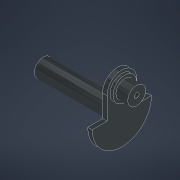
# Autodesk Inventor part: P015-Vilbrequin
Saved by Autodesk Inventor 2021.3 (Build 253353000, 353)
## iProperties
Created: 2022-04-01
Part Number: P015-Vilbrequin
Material: Iron, Gray
Document SubType Name: Modeling
Designer: remi
Density: 7.15 g/cm^3
Appearance: Iron Gray
Mass: 76.739 g
Surface Area: 54.5385 cm^2
Volume: 10.7327 cm^3
Author: remi
Autodesk Inventor part; units mm, degrees
ref_plane "YZ Plane" through (0, 0, 0) normal (1, 0, 0) x (0, 1, 0)
ref_plane "XZ Plane" through (0, 0, 0) normal (0, 1, 0) x (-1, 0, 0)
ref_plane "XY Plane" through (0, 0, 0) normal (0, 0, 1) x (1, 0, 0)
sketch "Sketch2" plane through (0, 0, 0) normal (1, 0, 0) x (0, 1, 0)
  arc A0 (-20, 0) -> (20, 0) centre (0, 0) ccw
  line L0 (-20, 0) -> (-10, 0)
  line L1 (-10, 0) -> (-10, 15)
  line L2 (20, 0) -> (10, 0)
  line L3 (10, 0) -> (10, 15)
  arc A1 (10, 15) -> (-10, 15) centre (0, 15) ccw
  dimension "d1" = 20
  dimension "d2" = 15
  dimension "d3" = 20
  constraints: 8 end point, 4 horizontal alignment, 4 point on circle, 2 centre point, 2 horizontal, 2 perpendicular, 1 coincident, 1 collinear
  measures "d1" distance between parallel lines of L3 L1
  measures "d2" distance of L2.end L3.end
  measures "d3" radius of A0
extrude "Extrusion1" add sketch "Sketch2" along normal blind 3
sketch "Sketch10" plane through (0, 0, 0) normal (-1, 0, 0) x (0, 0, 1)
  circle A0 centre (0, 0) radius 6
  dimension "d25" = 12
  constraints: 1 centre point, 1 coincident
  measures "d25" diameter of A0
extrude "Extrusion8" add sketch "Sketch10" along normal blind 50
sketch "Sketch11" plane through (3, 0, 0) normal (1, 0, 0) x (0, 0, -1)
  circle A0 centre (-15, 0) radius 6
  circle A1 centre (-15, 0) radius 8
  arc A2 (0, -20) -> (0, 20) centre (0, 0) ccw projected
  line L0 (0, 20) -> (0, 10) projected
  line L1 (0, 10) -> (-15, 10) projected
  arc A3 (-15, 10) -> (-15, -10) centre (-15, 0) ccw projected
  line L2 (-15, -10) -> (0, -10) projected
  line L3 (0, -10) -> (0, -20) projected
  dimension "d29" = 12
  dimension "d32" = 2
  constraints: 2 centre point, 2 coincident, 1 horizontal alignment
  measures "d29" diameter of A0
  measures "d32" radial gap between concentric circles of A1 A0
extrude "Extrusion9" add sketch "Sketch11" along normal blind 10 contours A0
extrude "Extrusion10" add sketch "Sketch11" along normal blind 2 contours A1
sketch "Sketch12" plane through (13, 0, 15) normal (1, 0, 0) x (0, 0, -1)
  circle A0 centre (0, 0) radius 6 construction
  point P0 (15, 0)
  constraints: 1 coincident
hole "Hole2" at (13, 0, 15) direction (-1, 0, 0) diameter 3.242 depth 10 tip angle 118 thread size "M4x0.7" class "6H" standard "ISO Metric profile"
body "Solid1"
